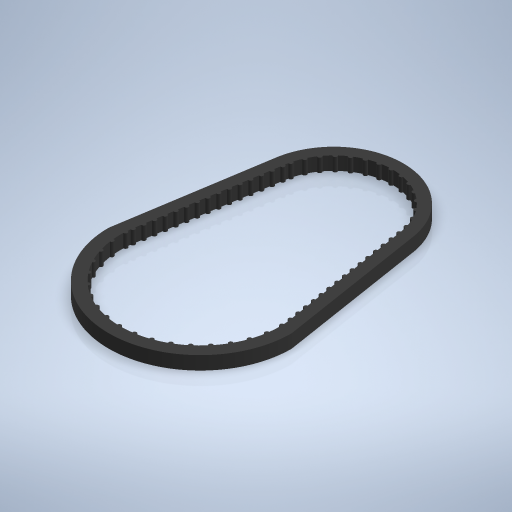
# Autodesk Inventor part: Belt
Saved by Autodesk Inventor 2024 (Build 280153000, 153)
## iProperties
Created: 2024-03-22
Part Number: Belt
Material: Gummi
Document SubType Name: Modeling
Designer: ffogue
Density: 0.93 g/cm^3
Appearance: Gummi - Schwarz
Author: ffogue
Autodesk Inventor part; units mm, degrees
ref_plane "XZ Plane" through (0, 0, 0) normal (0, 1, 0) x (-1, 0, 0)
sketch "Skizze1" plane through (0, 0, 0) normal (0, 0, 1) x (1, 0, 0)
  arc A0 (-294.5457, 46.6515) -> (294.5457, 46.6515) centre (0, 0) ccw
  arc A1 (217.2914, 534.4156) -> (-217.2914, 534.4156) centre (0, 500) ccw
  line L0 (-294.5457, 46.6515) -> (-217.2914, 534.4156)
  line L1 (294.5457, 46.6515) -> (217.2914, 534.4156)
  line L2 (0, 0) -> (0, 855.3898) construction
  arc A2 (-342.4332, 0) -> (342.4332, 0) centre (0, 0) ccw
  arc A3 (256.799, 540.673) -> (-256.799, 540.673) centre (0, 500) ccw
  line L3 (-342.4332, 0) -> (-256.799, 540.673)
  line L4 (256.799, 540.673) -> (342.4332, 0)
  dimension "d0" = 500
  dimension "d1" = 18
  dimension "d2" = 220
  dimension "d5" = 260
  constraints: 10 end point, 8 point on circle, 6 tangent, 4 centre point, 2 coincident, 2 concentric, 2 horizontal alignment, 2 symmetric about line, 1 parallel, 1 vertical, 1 vertical alignment
  measures "d0" distance of A0.centre A1.centre
  measures "d1" angle of L1 L0
  measures "d2" radius of A1
  measures "d5" radius of A3
extrude "Extrusion2" add sketch "Skizze1" along normal mid plane 50
sketch "Skizze2" plane through (-217.2914, 534.4156, 25) normal (0.9876883, -0.1564345, 0) x (0, 0, -1)
  line L0 (0, -493.8442) -> (0, 0) projected
  line L1 (50, 0) -> (50, -493.8442) projected
  line L2 (0, 0) -> (50, 0)
  line L3 (50, 0) -> (50, -15)
  line L4 (50, -15) -> (0, -15)
  line L5 (0, -15) -> (0, 0)
  line L6 (0, -493.8442) -> (50, -493.8442) projected
  line L7 (50, 0) -> (0, 0) projected
  point P0 (25, -493.8442)
  point P1 (0, -15)
  point P2 (25, 0)
  dimension "d9" = 15
  constraints: 8 end point, 2 midpoint, 2 parallel, 2 point on line, 1 horizontal, 1 perpendicular
  measures "d9" distance between parallel lines of L4 L2
extrude "Extrusion3" add sketch "Skizze2" along normal blind 8 contours L0 L2 L1 L4
fillet "Rundung1" radius 7.5 2 edges at (-209.3899, 533.1641, 0) (-211.7364, 518.3488, 0)
pattern_linear "Rechteckige Anordnung1" count 15 spacing 35 along (-0.1564345, -0.9876883, 0) of "Rundung1", "Extrusion3"
ref_plane "Arbeitsebene1" through (0, 0, 0) normal (1, 0, 0) x (0, 1, 0)
mirror "Spiegeln4" about plane through (0, 0, 0) normal (1, 0, 0) of "Rundung1", "Extrusion3", "Rechteckige Anordnung1"
fillet "Rundung2" radius 50 1 edges at (342.4332, 0, 0)
fillet "Rundung3" radius 50 1 edges at (-342.4332, 0, 0)
ref_plane "Arbeitsebene3" through (0, 0, -25) normal (0, 0, -1) x (-1, 0, 0)
sketch "Skizze4" plane through (0, 0, -25) normal (0, 0, -1) x (-1, 0, 0)
  arc A0 (217.2914, 534.4156) -> (-217.2914, 534.4156) centre (0, 500) ccw projected
  line L0 (-222.7666, 499.8465) -> (-219.638, 519.6003) projected
  arc A1 (-219.1441, 519.522) -> (-216.7976, 534.3374) centre (-217.9708, 526.9297) ccw projected
  arc A2 (-224.6193, 484.9529) -> (-222.2728, 499.7683) centre (-223.4461, 492.3606) ccw projected
  arc A3 (-213.2574, 554.0487) -> (-209.0794, 568.4528) centre (-211.2912, 561.2864) ccw
  point P0 (0, 0)
  dimension "d29" = 35
  dimension "d30" = 7.5
  constraints: 5 point on circle, 1 centre point
  measures "d29" distance of A1.centre A3.centre
  measures "d30" radius of A3
extrude "Extrusion5" add sketch "Skizze4" against normal up to surface (50 mm away)
pattern_circular "Runde Anordnung2" count 15 over 150 about axis through (0, 500, 0) along (0, 0, 1) of "Extrusion5"
sketch "Skizze5" plane through (0, 0, -25) normal (0, 0, -1) x (-1, 0, 0)
  arc A0 (-296.0847, 35.6003) -> (296.0847, 35.6003) centre (0, 0) ccw projected
  arc A1 (-298.2169, 0.4632) -> (-297.8164, 15.4566) centre (-298.1109, 7.9624) ccw
  arc A2 (-295.797, 35.5548) -> (-293.4505, 50.3701) centre (-294.6237, 42.9624) ccw projected
  point P0 (294.5457, 46.6515)
  point P1 (-294.5457, 46.6515)
  dimension "d36" = 7.5
  dimension "d37" = 35
  constraints: 5 point on circle, 1 centre point
  measures "d36" radius of A1
  measures "d37" vertical distance of A1.centre A2.centre
extrude "Extrusion6" add sketch "Skizze5" against normal up to surface (50 mm away)
pattern_circular "Runde Anordnung3" count 19 over 185 about axis through (0, 0, 0) along (0, 0, -1) of "Extrusion6"
